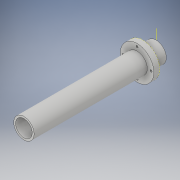
# Autodesk Inventor part: waveguide
Saved by Autodesk Inventor 2017 (Build 210142000, 142)
## iProperties
Created: 2017-06-22
Part Number: waveguide
Material: Generic
Document SubType Name: Modeling
Designer: Zara
Density: 1 g/cm^3
Appearance: Default
Author: Zara
Autodesk Inventor part; units mm, degrees
ref_plane "YZ Plane" through (0, 0, 0) normal (1, 0, 0) x (0, 1, 0)
ref_plane "XZ Plane" through (0, 0, 0) normal (0, 1, 0) x (-1, 0, 0)
ref_plane "XY Plane" through (0, 0, 0) normal (0, 0, 1) x (1, 0, 0)
sketch "Sketch1" plane through (0, 0, 0) normal (0, 0, 1) x (1, 0, 0)
  circle A0 centre (0, 0) radius 6.2865
  circle A1 centre (0, 0) radius 7.7343
  circle A2 centre (0, 0) radius 12.7
  dimension "d0" = 12.573
  dimension "d1" = 15.4686
  dimension "d4" = 25.4
  constraints: 3 centre point, 3 coincident
  measures "d0" diameter of A0
  measures "d1" diameter of A1
  measures "d4" diameter of A2
extrude "Extrusion2" add sketch "Sketch1" along normal blind 100 contours A1 | A2
extrude "Extrusion3" cut sketch "Sketch1" along normal blind 10.0076 contours A2
sketch "Sketch3" plane through (0, 0, 100) normal (0, 0, 1) x (1, 0, 0)
  circle A0 centre (0, 0) radius 12.7 projected
  circle A1 centre (0, 0) radius 7.7343 projected
  circle A2 centre (0, 0) radius 6.2865 projected
  circle A3 centre (0, 0) radius 6.2865 projected
  circle A4 centre (0, 0) radius 6.2865 projected
extrude "Extrusion4" cut sketch "Sketch3" against normal blind 85.598 contours A0
sketch "Sketch4" plane through (0, 0, 10.0076) normal (0, 0, -1) x (-1, 0, 0)
  circle A0 centre (0, 0) radius 10.6045 construction
  point P0 (0, 10.6045)
  point P1 (0, -10.6045)
  point P2 (-10.6045, 0)
  point P3 (10.6045, 0)
  dimension "d11" = 21.209
  constraints: 4 point on circle, 1 centre point, 1 coincident
  measures "d11" diameter of A0
hole "Hole1" at (0, 10.6045, 10.0076) at (10.6045, 0, 10.0076) at (-10.6045, 0, 10.0076) at (0, -10.6045, 10.0076) direction (0, 0, 1) diameter 1.5748 depth 6.2992 tip angle 118
sketch "Sketch5" plane through (0, 0, 10.0076) normal (0, 0, -1) x (-1, 0, 0)
  point P0 (0, 0)
sketch "Sketch6" plane through (0, 0, 10.0076) normal (0, 0, -1) x (-1, 0, 0)
  circle A0 centre (0, 10.6045) radius 0.7874 construction
  line L0 (0, 10.6045) -> (0, 12.7) construction
  circle A1 centre (0, 0) radius 12.7 construction
  constraints: 2 end point, 1 vertical, 1 vertical alignment, 1 other
body "Solid2"
